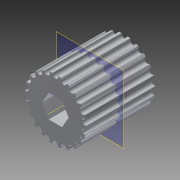
# Autodesk Inventor part: 22T 5mm GT2 - .500 Hex Broach
Saved by Autodesk Inventor 2013 (Build 170138000, 138)
## iProperties
Created: 2013-06-25
Part Number: 22T 5mm GT2 - .500 Hex Broach
Material: Generic
Document SubType Name: Modeling
Designer: mvarma
Density: 1 g/cm^3
Author: mvarma
Autodesk Inventor part; units mm, degrees
ref_plane "YZ Plane" through (0, 0, 0) normal (1, 0, 0) x (0, 1, 0)
ref_plane "XZ Plane" through (0, 0, 0) normal (0, 1, 0) x (-1, 0, 0)
ref_plane "XY Plane" through (0, 0, 0) normal (0, 0, 1) x (1, 0, 0)
sketch "Sketch1" plane through (0, 0, 0) normal (0, 0, 1) x (1, 0, 0)
  arc A0 (-1.4681, -0.0864) -> (1.4681, -0.0864) centre (0, 0) ccw
  arc A1 (-1.4681, -0.0864) -> (-1.4773, 0) centre (-2.3809, -0.1401) ccw
  arc A2 (-1.4773, 0) -> (-1.7414, 0.4234) centre (-2.1048, -0.0973) ccw
  arc A3 (-1.7414, 0.4234) -> (-3.0806, 0.2309) centre (0, -16.4419) ccw
  arc A4 (-3.0806, 0.2309) -> (-3.2147, -0.2498) centre (-2.5852, -0.1664) ccw
  arc A5 (-3.2147, -0.2498) -> (-3.1992, -0.3353) centre (-2.3083, -0.1297) ccw
  arc A6 (-6.0165, -1.1625) -> (-3.1992, -0.3353) centre (-4.6322, -0.666) ccw
  arc A7 (-6.0165, -1.1625) -> (-6.0497, -1.0822) centre (-6.8772, -1.4712) ccw
  arc A8 (-6.0497, -1.0822) -> (-6.4224, -0.7504) centre (-6.6244, -1.3524) ccw
  arc A9 (-6.4224, -0.7504) -> (-7.6531, -1.3124) centre (0, -16.4419) ccw
  arc A10 (-7.6531, -1.3124) -> (-7.6464, -1.8114) centre (-7.0659, -1.554) ccw
  arc A11 (-7.6464, -1.8114) -> (-7.6074, -1.8891) centre (-6.8104, -1.4407) ccw
  arc A12 (-10.0775, -3.4765) -> (-7.6074, -1.8891) centre (-8.8892, -2.6101) ccw
  arc A13 (-10.0775, -3.4765) -> (-10.132, -3.4088) centre (-10.8164, -4.0152) ccw
  arc A14 (-10.132, -3.4088) -> (-10.5831, -3.1954) centre (-10.6073, -3.8299) ccw
  arc A15 (-10.5831, -3.1954) -> (-11.6056, -4.0814) centre (0, -16.4419) ccw
  arc A16 (-11.6056, -4.0814) -> (-11.4585, -4.5583) centre (-10.9741, -4.1477) ccw
  arc A17 (-11.4585, -4.5583) -> (-11.3993, -4.6218) centre (-10.7609, -3.9671) ccw
  arc A18 (-13.3221, -6.8409) -> (-11.3993, -4.6218) centre (-12.426, -5.6748) ccw
  arc A19 (-13.3221, -6.8409) -> (-13.3934, -6.7913) centre (-13.8793, -7.5659) ccw
  arc A20 (-13.3934, -6.7913) -> (-13.8864, -6.7135) centre (-13.7308, -7.3292) ccw
  arc A21 (-13.8864, -6.7135) -> (-14.6178, -7.8518) centre (0, -16.4419) ccw
  arc A22 (-14.6178, -7.8518) -> (-14.3424, -8.2679) centre (-13.9932, -7.7375) ccw
  arc A23 (-14.3424, -8.2679) -> (-14.2676, -8.3121) centre (-13.8396, -7.5041) ccw
  arc A24 (-15.4874, -10.983) -> (-14.2676, -8.3121) centre (-14.9561, -9.6117) ccw
  arc A25 (-15.4874, -10.983) -> (-15.5698, -10.9555) centre (-15.8177, -11.8357) ccw
  arc A26 (-15.5698, -10.9555) -> (-16.0647, -11.0199) centre (-15.742, -11.5668) ccw
  arc A27 (-16.0647, -11.0199) -> (-16.4458, -12.318) centre (0, -16.4419) ccw
  arc A28 (-16.4458, -12.318) -> (-16.0643, -12.6397) centre (-15.8787, -12.0324) ccw
  arc A29 (-16.0643, -12.6397) -> (-15.9801, -12.6611) centre (-15.797, -11.7652) ccw
  arc A30 (-16.398, -15.5675) -> (-15.9801, -12.6611) centre (-16.2746, -14.102) ccw
  arc A31 (-16.398, -15.5675) -> (-16.4848, -15.5643) centre (-16.4747, -16.4786) ccw
  arc A32 (-16.4848, -15.5643) -> (-16.9415, -15.7654) centre (-16.4778, -16.1993) ccw
  arc A33 (-16.9415, -15.7654) -> (-16.9415, -17.1184) centre (0, -16.4419) ccw
  arc A34 (-16.9415, -17.1184) -> (-16.4848, -17.3195) centre (-16.4778, -16.6846) ccw
  arc A35 (-16.4848, -17.3195) -> (-16.398, -17.3164) centre (-16.4747, -16.4052) ccw
  arc A36 (-15.9801, -20.2227) -> (-16.398, -17.3164) centre (-16.2746, -18.7818) ccw
  arc A37 (-15.9801, -20.2227) -> (-16.0643, -20.2442) centre (-15.797, -21.1186) ccw
  arc A38 (-16.0643, -20.2442) -> (-16.4458, -20.5658) centre (-15.8787, -20.8514) ccw
  arc A39 (-16.4458, -20.5658) -> (-16.0647, -21.864) centre (0, -16.4419) ccw
  arc A40 (-16.0647, -21.864) -> (-15.5698, -21.9283) centre (-15.742, -21.3171) ccw
  arc A41 (-15.5698, -21.9283) -> (-15.4874, -21.9008) centre (-15.8177, -21.0482) ccw
  arc A42 (-14.2676, -24.5717) -> (-15.4874, -21.9008) centre (-14.9561, -23.2721) ccw
  arc A43 (-14.2676, -24.5717) -> (-14.3424, -24.616) centre (-13.8396, -25.3797) ccw
  arc A44 (-14.3424, -24.616) -> (-14.6178, -25.0321) centre (-13.9932, -25.1463) ccw
  arc A45 (-14.6178, -25.0321) -> (-13.8864, -26.1703) centre (0, -16.4419) ccw
  arc A46 (-13.8864, -26.1703) -> (-13.3934, -26.0926) centre (-13.7308, -25.5546) ccw
  arc A47 (-13.3934, -26.0926) -> (-13.3221, -26.043) centre (-13.8793, -25.3179) ccw
  arc A48 (-11.3993, -28.262) -> (-13.3221, -26.043) centre (-12.426, -27.2091) ccw
  arc A49 (-11.3993, -28.262) -> (-11.4585, -28.3256) centre (-10.7609, -28.9167) ccw
  arc A50 (-11.4585, -28.3256) -> (-11.6056, -28.8024) centre (-10.9741, -28.7361) ccw
  arc A51 (-11.6056, -28.8024) -> (-10.5831, -29.6885) centre (0, -16.4419) ccw
  arc A52 (-10.5831, -29.6885) -> (-10.132, -29.475) centre (-10.6073, -29.0539) ccw
  arc A53 (-10.132, -29.475) -> (-10.0775, -29.4073) centre (-10.8164, -28.8686) ccw
  arc A54 (-7.6074, -30.9948) -> (-10.0775, -29.4073) centre (-8.8892, -30.2737) ccw
  arc A55 (-7.6074, -30.9948) -> (-7.6464, -31.0725) centre (-6.8104, -31.4431) ccw
  arc A56 (-7.6464, -31.0725) -> (-7.6531, -31.5714) centre (-7.0659, -31.3298) ccw
  arc A57 (-7.6531, -31.5714) -> (-6.4224, -32.1335) centre (0, -16.4419) ccw
  arc A58 (-6.4224, -32.1335) -> (-6.0497, -31.8016) centre (-6.6244, -31.5315) ccw
  arc A59 (-6.0497, -31.8016) -> (-6.0165, -31.7213) centre (-6.8772, -31.4126) ccw
  arc A60 (-3.1992, -32.5485) -> (-6.0165, -31.7213) centre (-4.6322, -32.2178) ccw
  arc A61 (-3.1992, -32.5485) -> (-3.2147, -32.634) centre (-2.3083, -32.7542) ccw
  arc A62 (-3.2147, -32.634) -> (-3.0806, -33.1147) centre (-2.5852, -32.7175) ccw
  arc A63 (-3.0806, -33.1147) -> (-1.7414, -33.3073) centre (0, -16.4419) ccw
  arc A64 (-1.7414, -33.3073) -> (-1.4773, -32.8838) centre (-2.1048, -32.7865) ccw
  arc A65 (-1.4773, -32.8838) -> (-1.4681, -32.7974) centre (-2.3809, -32.7437) ccw
  arc A66 (1.4681, -32.7974) -> (-1.4681, -32.7974) centre (0, -32.8838) ccw
  arc A67 (1.4681, -32.7974) -> (1.4773, -32.8838) centre (2.3809, -32.7437) ccw
  arc A68 (1.4773, -32.8838) -> (1.7414, -33.3073) centre (2.1048, -32.7865) ccw
  arc A69 (1.7414, -33.3073) -> (3.0806, -33.1147) centre (0, -16.4419) ccw
  arc A70 (3.0806, -33.1147) -> (3.2147, -32.634) centre (2.5852, -32.7175) ccw
  arc A71 (3.2147, -32.634) -> (3.1992, -32.5485) centre (2.3083, -32.7542) ccw
  arc A72 (6.0165, -31.7213) -> (3.1992, -32.5485) centre (4.6322, -32.2178) ccw
  arc A73 (6.0165, -31.7213) -> (6.0497, -31.8016) centre (6.8772, -31.4126) ccw
  arc A74 (6.0497, -31.8016) -> (6.4224, -32.1335) centre (6.6244, -31.5315) ccw
  arc A75 (6.4224, -32.1335) -> (7.6531, -31.5714) centre (0, -16.4419) ccw
  arc A76 (7.6531, -31.5714) -> (7.6464, -31.0725) centre (7.0659, -31.3298) ccw
  arc A77 (7.6464, -31.0725) -> (7.6074, -30.9948) centre (6.8104, -31.4431) ccw
  arc A78 (10.0775, -29.4073) -> (7.6074, -30.9948) centre (8.8892, -30.2737) ccw
  arc A79 (10.0775, -29.4073) -> (10.132, -29.475) centre (10.8164, -28.8686) ccw
  arc A80 (10.132, -29.475) -> (10.5831, -29.6885) centre (10.6073, -29.0539) ccw
  arc A81 (10.5831, -29.6885) -> (11.6056, -28.8024) centre (0, -16.4419) ccw
  arc A82 (11.6056, -28.8024) -> (11.4585, -28.3256) centre (10.9741, -28.7361) ccw
  arc A83 (11.4585, -28.3256) -> (11.3993, -28.262) centre (10.7609, -28.9167) ccw
  arc A84 (13.3221, -26.043) -> (11.3993, -28.262) centre (12.426, -27.2091) ccw
  arc A85 (13.3221, -26.043) -> (13.3934, -26.0926) centre (13.8793, -25.3179) ccw
  arc A86 (13.3934, -26.0926) -> (13.8864, -26.1703) centre (13.7308, -25.5546) ccw
  arc A87 (13.8864, -26.1703) -> (14.6178, -25.0321) centre (0, -16.4419) ccw
  arc A88 (14.6178, -25.0321) -> (14.3424, -24.616) centre (13.9932, -25.1463) ccw
  arc A89 (14.3424, -24.616) -> (14.2676, -24.5717) centre (13.8396, -25.3797) ccw
  arc A90 (15.4874, -21.9008) -> (14.2676, -24.5717) centre (14.9561, -23.2721) ccw
  arc A91 (15.4874, -21.9008) -> (15.5698, -21.9283) centre (15.8177, -21.0482) ccw
  arc A92 (15.5698, -21.9283) -> (16.0647, -21.864) centre (15.742, -21.3171) ccw
  arc A93 (16.0647, -21.864) -> (16.4458, -20.5658) centre (0, -16.4419) ccw
  arc A94 (16.4458, -20.5658) -> (16.0643, -20.2442) centre (15.8787, -20.8514) ccw
  arc A95 (16.0643, -20.2442) -> (15.9801, -20.2227) centre (15.797, -21.1186) ccw
  arc A96 (16.398, -17.3164) -> (15.9801, -20.2227) centre (16.2746, -18.7818) ccw
  arc A97 (16.398, -17.3164) -> (16.4848, -17.3195) centre (16.4747, -16.4052) ccw
  arc A98 (16.4848, -17.3195) -> (16.9415, -17.1184) centre (16.4778, -16.6846) ccw
  arc A99 (16.9415, -17.1184) -> (16.9415, -15.7654) centre (0, -16.4419) ccw
  arc A100 (16.9415, -15.7654) -> (16.4848, -15.5643) centre (16.4778, -16.1993) ccw
  arc A101 (16.4848, -15.5643) -> (16.398, -15.5675) centre (16.4747, -16.4786) ccw
  arc A102 (15.9801, -12.6611) -> (16.398, -15.5675) centre (16.2746, -14.102) ccw
  arc A103 (15.9801, -12.6611) -> (16.0643, -12.6397) centre (15.797, -11.7652) ccw
  arc A104 (16.0643, -12.6397) -> (16.4458, -12.318) centre (15.8787, -12.0324) ccw
  arc A105 (16.4458, -12.318) -> (16.0647, -11.0199) centre (0, -16.4419) ccw
  arc A106 (16.0647, -11.0199) -> (15.5698, -10.9555) centre (15.742, -11.5668) ccw
  arc A107 (15.5698, -10.9555) -> (15.4874, -10.983) centre (15.8177, -11.8357) ccw
  arc A108 (14.2676, -8.3121) -> (15.4874, -10.983) centre (14.9561, -9.6117) ccw
  arc A109 (14.2676, -8.3121) -> (14.3424, -8.2679) centre (13.8396, -7.5041) ccw
  arc A110 (14.3424, -8.2679) -> (14.6178, -7.8518) centre (13.9932, -7.7375) ccw
  arc A111 (14.6178, -7.8518) -> (13.8864, -6.7135) centre (0, -16.4419) ccw
  arc A112 (13.8864, -6.7135) -> (13.3934, -6.7913) centre (13.7308, -7.3292) ccw
  arc A113 (13.3934, -6.7913) -> (13.3221, -6.8409) centre (13.8793, -7.5659) ccw
  arc A114 (11.3993, -4.6218) -> (13.3221, -6.8409) centre (12.426, -5.6748) ccw
  arc A115 (11.3993, -4.6218) -> (11.4585, -4.5583) centre (10.7609, -3.9671) ccw
  arc A116 (11.4585, -4.5583) -> (11.6056, -4.0814) centre (10.9741, -4.1477) ccw
  arc A117 (11.6056, -4.0814) -> (10.5831, -3.1954) centre (0, -16.4419) ccw
  arc A118 (10.5831, -3.1954) -> (10.132, -3.4088) centre (10.6073, -3.8299) ccw
  arc A119 (10.132, -3.4088) -> (10.0775, -3.4765) centre (10.8164, -4.0152) ccw
  arc A120 (7.6074, -1.8891) -> (10.0775, -3.4765) centre (8.8892, -2.6101) ccw
  arc A121 (7.6074, -1.8891) -> (7.6464, -1.8114) centre (6.8104, -1.4407) ccw
  arc A122 (7.6464, -1.8114) -> (7.6531, -1.3124) centre (7.0659, -1.554) ccw
  arc A123 (7.6531, -1.3124) -> (6.4224, -0.7504) centre (0, -16.4419) ccw
  arc A124 (6.4224, -0.7504) -> (6.0497, -1.0822) centre (6.6244, -1.3524) ccw
  arc A125 (6.0497, -1.0822) -> (6.0165, -1.1625) centre (6.8772, -1.4712) ccw
  arc A126 (3.1992, -0.3353) -> (6.0165, -1.1625) centre (4.6322, -0.666) ccw
  arc A127 (3.1992, -0.3353) -> (3.2147, -0.2498) centre (2.3083, -0.1297) ccw
  arc A128 (3.2147, -0.2498) -> (3.0806, 0.2309) centre (2.5852, -0.1664) ccw
  arc A129 (3.0806, 0.2309) -> (1.7414, 0.4234) centre (0, -16.4419) ccw
  arc A130 (1.7414, 0.4234) -> (1.4773, 0) centre (2.1048, -0.0973) ccw
  arc A131 (1.4773, 0) -> (1.4681, -0.0864) centre (2.3809, -0.1401) ccw
  line L0 (-7.3323, -16.4419) -> (-3.6662, -10.0919)
  line L1 (-3.6662, -10.0919) -> (3.6662, -10.0919)
  line L2 (3.6662, -10.0919) -> (7.3323, -16.4419)
  line L3 (7.3323, -16.4419) -> (3.6662, -22.7919)
  line L4 (3.6662, -22.7919) -> (-3.6662, -22.7919)
  line L5 (-3.6662, -22.7919) -> (-7.3323, -16.4419)
  dimension "d0" = 12.7
  constraints: 264 point on circle, 132 centre point, 12 end point, 1 coincident, 1 horizontal, 410 other
  measures "d0" distance between parallel lines of L4 L1
extrude "Extrusion1" add sketch "Sketch1" along normal blind 38.1
ref_plane "Work Plane1" through (0, 0, 19.05) normal (0, 0, -1) x (-1, 0, 0)
body "Solid1"
